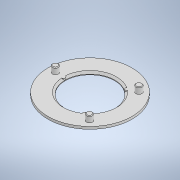
# Autodesk Inventor part: Шапка лидара
Saved by Autodesk Inventor 2020 (Build 240168000, 168)
## iProperties
Created: 2021-08-20
Part Number: Шапка лидара
Material: Типовые
Document SubType Name: Modeling
Designer: Антон
Density: 1 g/cm^3
Appearance: По умолчанию
Author: Антон
Autodesk Inventor part; units mm, degrees
ref_plane "YZ Plane" through (0, 0, 0) normal (1, 0, 0) x (0, 1, 0)
ref_plane "XZ Plane" through (0, 0, 0) normal (0, 1, 0) x (-1, 0, 0)
ref_plane "XY Plane" through (0, 0, 0) normal (0, 0, 1) x (1, 0, 0)
sketch "Эскиз1" plane through (0, 0, 0) normal (0, 1, 0) x (-1, 0, 0)
  circle A0 centre (0, 0) radius 34
  dimension "d0" = 68
  constraints: 1 centre point, 1 coincident
  measures "d0" diameter of A0
extrude "Выдавливание1" add sketch "Эскиз1" along normal blind 2
sketch "Эскиз2" plane through (0, 2, 0) normal (0, 1, 0) x (1, 0, 0)
  circle A0 centre (0, 0) radius 28
  line L0 (19.5959, -20) -> (19.5959, 20)
  line L1 (19.5959, -20) -> (-28, 0)
  line L2 (19.5959, 20) -> (-28, 0)
  circle A1 centre (-28, 0) radius 2.5
  circle A2 centre (19.5959, -20) radius 2.5
  circle A3 centre (19.5959, 20) radius 2.5
  dimension "d3" = 56
  dimension "d4" = 40
  dimension "d5" = 5
  constraints: 6 end point, 4 centre point, 4 coincident, 3 point on circle, 2 equal radius, 1 equal length, 1 vertical
  measures "d3" diameter of A0
  measures "d4" distance of L0.start L0.end
  measures "d5" diameter of A1
extrude "Выдавливание2" add sketch "Эскиз2" along normal blind 5 contours A3 L0 A0 | A0 A3 | A2 A0 | A0 L0 A2 | L2 A3 A0 | L0 A3 L2 | L1 A2 L0 | A0 A2 L1 | A1 L2 A0 | A0 A1 | A1 L1 L2 | A0 L1 A1
chamfer "Фаска1" distance 0.5 angle 45 3 edges at (17.0959, 7, -20) (17.0959, 7, 20) (-30.5, 7, 0)
sketch "Эскиз3" plane through (0, 2, 0) normal (0, 1, 0) x (1, 0, 0)
  circle A0 centre (0, 0) radius 20
  circle A1 centre (-28, 0) radius 2 projected
  circle A2 centre (19.5959, 20) radius 2 projected
  circle A3 centre (19.5959, -20) radius 2 projected
  line L0 (-28, 0) -> (19.5959, -20)
  circle A4 centre (-28, 0) radius 2.5 projected
  line L1 (19.5959, 20) -> (-28, 0)
  circle A5 centre (11.289, -16.5094) radius 1.5
  circle A6 centre (11.289, 16.5094) radius 1.5
  circle A7 centre (-20, 0) radius 1.5
  dimension "d11" = 40
  dimension "d17" = 3
  constraints: 4 centre point, 4 end point, 3 point on circle, 2 equal radius, 2 point on line, 1 coincident, 1 horizontal alignment
  measures "d11" diameter of A0
  measures "d17" diameter of A5
extrude "Выдавливание3" cut sketch "Эскиз3" against normal blind 5 contours A0 A5 L0 A7 L1 A6 | A6 L1 A0 | A0 L0 A5 | L1 A6 A0 | L1 A0 A6 | A0 A5 L0 | A5 A0 L0 | A7 A0 picked at (11.3081, 15.9275) picked at (11.3081, -15.9275) picked at (10.6892, 16.4081) picked at (-9.3619, 9.1636) picked at (10.6892, -16.4081) picked at (-9.3619, -9.1636) picked at (-19.4958, 0)
chamfer "Фаска2" distance 1.5 angle 45 1 edges at (-20, 2, 0)
sketch "Эскиз4" plane through (0, 2, 0) normal (0, 1, 0) x (1, 0, 0)
  circle A0 centre (-28, 0) radius 2 projected
  circle A1 centre (19.5959, -20) radius 2 projected
  circle A2 centre (19.5959, 20) radius 2 projected
  circle A3 centre (-28, 0) radius 2 projected
  line L0 (19.5959, -20) -> (-28, 0)
  circle A4 centre (19.5959, 20) radius 2 projected
  line L1 (-28, 0) -> (19.5959, 20)
  circle A5 centre (0, 0) radius 20 projected
  circle A6 centre (0, 0) radius 21.5 projected
  circle A7 centre (12.9117, 17.1912) radius 1.5
  circle A8 centre (12.9117, -17.1912) radius 1.5
  circle A9 centre (-21.5, 0) radius 1.5
  constraints: 4 end point, 3 centre point, 3 point on circle, 3 tangent, 2 point on line, 1 horizontal alignment
extrude "Выдавливание4" add sketch "Эскиз4" against normal up to surface (2 mm away) contours A7 L1 A6 | A6 L1 A7 | A9 A6 | A6 A9 | A8 L0 A6 | A6 L0 A8 | A6 A7 L1 | L1 A7 A6 | A6 A8 L0 | L0 A8 A6
